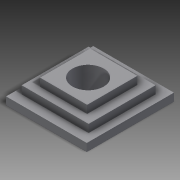
# Autodesk Inventor part: 1st part ever
Saved by Autodesk Inventor 2015 (Build 190159000, 159)
## iProperties
Created: 2015-08-29
Part Number: 1st part ever
Material: Generic
Document SubType Name: Modeling
Designer: Brandon
Density: 1 g/cm^3
Appearance: Default
Author: Brandon
Autodesk Inventor part; units mm, degrees
ref_plane "YZ Plane" through (0, 0, 0) normal (1, 0, 0) x (0, 1, 0)
ref_plane "XZ Plane" through (0, 0, 0) normal (0, 1, 0) x (-1, 0, 0)
ref_plane "XY Plane" through (0, 0, 0) normal (0, 0, 1) x (1, 0, 0)
sketch "Sketch5" plane through (0, 0, 0) normal (0, 1, 0) x (-1, 0, 0)
  line L0 (27.9234, 26.0727) -> (-26.467, 26.0727)
  line L1 (-26.467, 26.0727) -> (-26.467, -28.3178)
  line L2 (-26.467, -28.3178) -> (27.9234, -28.3178)
  line L3 (27.9234, -28.3178) -> (27.9234, 26.0727)
  point P0 (0, 0)
  constraints: 8 end point, 2 parallel, 1 horizontal, 1 perpendicular
extrude "Extrusion3" add sketch "Sketch5" along normal blind 6.35
sketch "Sketch6" plane through (0, 0, 0) normal (0, -1, 0) x (1, 0, 0)
  line L0 (-32.7834, 33.8762) -> (32.7834, 33.8762)
  line L1 (32.7834, 33.8762) -> (32.7834, -36.936)
  line L2 (32.7834, -36.936) -> (-32.7834, -36.936)
  line L3 (-32.7834, -36.936) -> (-32.7834, 33.8762)
  point P0 (0, 0)
  constraints: 8 end point, 2 parallel, 1 horizontal, 1 perpendicular
extrude "Extrusion4" add sketch "Sketch6" along normal blind 6.35
sketch "Sketch7" plane through (0, 6.35, 0) normal (0, 1, 0) x (1, 0, 0)
  line L0 (-19.5244, 21.2) -> (18.7958, 21.2)
  line L1 (18.7958, 21.2) -> (18.7958, -19.5972)
  line L2 (18.7958, -19.5972) -> (-19.5244, -19.5972)
  line L3 (-19.5244, -19.5972) -> (-19.5244, 21.2)
  point P0 (0, 0)
  constraints: 8 end point, 2 parallel, 1 horizontal, 1 perpendicular
extrude "Extrusion5" add sketch "Sketch7" along normal blind 6.35
sketch "Sketch8" plane through (0, 12.7, 0) normal (0, 1, 0) x (1, 0, 0)
  circle A0 centre (0, 0) radius 8.1896
  constraints: 1 centre point, 1 coincident
hole "Hole1" at (0, 12.7, 0) direction (0, -1, 0) diameter 25.4 end through all
body "Solid3"
